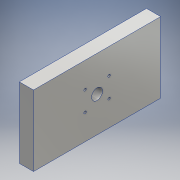
# Autodesk Inventor part: plate
Saved by Autodesk Inventor 2016 (Build 200138000, 138)
## iProperties
Created: 2016-07-15
Part Number: plate
Material: Aluminum 6061
Document SubType Name: Modeling
Designer: Jonathan
Density: 2.7 g/cm^3
Appearance: Aluminum - Flat
Author: Jonathan
Autodesk Inventor part; units mm, degrees
ref_plane "YZ Plane" through (0, 0, 0) normal (1, 0, 0) x (0, 1, 0)
ref_plane "XZ Plane" through (0, 0, 0) normal (0, 1, 0) x (-1, 0, 0)
ref_plane "XY Plane" through (0, 0, 0) normal (0, 0, 1) x (1, 0, 0)
sketch "Sketch1" plane through (0, 0, 0) normal (1, 0, 0) x (0, 1, 0)
  line L0 (57.15, 31.75) -> (-57.15, 31.75)
  line L1 (-57.15, 31.75) -> (-57.15, -31.75)
  line L2 (-57.15, -31.75) -> (57.15, -31.75)
  line L3 (57.15, -31.75) -> (57.15, 31.75)
  line L4 (-50.8, 25.4) -> (50.8, 25.4)
  line L5 (50.8, 25.4) -> (50.8, -25.4)
  line L6 (50.8, -25.4) -> (-50.8, -25.4)
  line L7 (-50.8, -25.4) -> (-50.8, 25.4)
  point P0 (0, 0)
  point P1 (0, -31.75)
  point P2 (57.15, 0)
  point P3 (0, 25.4)
  point P4 (-50.8, 0)
  dimension "d0" = 63.5
  dimension "d1" = 114.3
  dimension "d14" = 50.8
  dimension "d15" = 101.6
  constraints: 16 end point, 4 midpoint, 4 parallel, 2 horizontal, 2 horizontal alignment, 2 perpendicular, 2 vertical alignment
  measures "d0" distance of L2.end L0.start
  measures "d1" distance of L1.end L2.end
  measures "d14" distance of L4.end L5.end
  measures "d15" distance of L5.end L6.end
extrude "Extrusion1" add sketch "Sketch1" along normal blind 12.7 contours L3 L2 L1 L0 | L4 L5 L6 L7
sketch "Sketch2" plane through (12.7, 0, 0) normal (1, 0, 0) x (0, 0, -1)
  line L0 (-8.89, -10.795) -> (8.89, 10.795) construction
  line L1 (-8.89, 10.795) -> (8.89, -10.795) construction
  circle A0 centre (0, 0) radius 4.9609
  dimension "d5" = 21.59
  dimension "d12" = 9.9219
  dimension "d13" = 17.78
  constraints: 4 end point, 2 coincident, 2 horizontal alignment, 2 vertical alignment, 1 centre point, 1 midpoint
  measures "d5" distance of L1.start L0.start
  measures "d12" diameter of A0
  measures "d13" distance of L1.end L0.start
sketch "Sketch3" plane through (0, 0, 0) normal (-1, 0, 0) x (0, 0, 1)
  line L0 (-28.575, -53.975) -> (28.575, -53.975)
  line L1 (28.575, -53.975) -> (28.575, 53.975)
  line L2 (28.575, 53.975) -> (-28.575, 53.975)
  line L3 (-28.575, 53.975) -> (-28.575, -53.975)
  line L4 (22.098, 47.498) -> (22.098, -47.498)
  line L5 (22.098, -47.498) -> (-22.098, -47.498)
  line L6 (-22.098, -47.498) -> (-22.098, 47.498)
  line L7 (-22.098, 47.498) -> (22.098, 47.498)
  point P0 (0, 0)
  point P1 (0, -53.975)
  point P2 (-28.575, 0)
  point P3 (0, 0)
  point P4 (28.575, 0)
  point P5 (0, 53.975)
  dimension "d16" = 107.95
  dimension "d17" = 57.15
  dimension "d31" = 6.477
  constraints: 16 end point, 4 midpoint, 4 parallel, 2 horizontal alignment, 2 perpendicular, 1 coincident, 1 horizontal, 1 vertical alignment, 3 other
  measures "d16" distance of L2.end L0.start
  measures "d17" distance of L1.end L2.end
  measures "d31" distance between parallel lines of L1 L4
extrude "Extrusion3" cut sketch "Sketch3" against normal blind 3.175
extrude "Extrusion4" cut sketch "Sketch2" against normal through all
hole "Hole1" at (12.7, -10.795, 8.89) at (12.7, 10.795, 8.89) at (12.7, 10.795, -8.89) at (12.7, -10.795, -8.89) direction (-1, 0, 0) diameter 2.159 depth 8.8646 tip angle 118
fillet "Fillet1" radius 3.175 8 edges at (1.5875, 53.975, 28.575) (1.5875, -47.498, 22.098) (1.5875, -47.498, -22.098) (1.5875, -53.975, -28.575) (1.5875, 47.498, -22.098) (1.5875, -53.975, 28.575) (1.5875, 53.975, -28.575) (1.5875, 47.498, 22.098)
body "Solid1"
